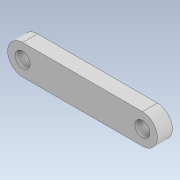
# Autodesk Inventor part: 地桿
Saved by Autodesk Inventor 2022 (Build 260153000, 153)
## iProperties
Created: 2023-05-12
Part Number: 地桿
Material: 一般
Document SubType Name: Modeling
Designer: JOU
Density: 1 g/cm^3
Appearance: 預設
Author: JOU
Autodesk Inventor part; units mm, degrees
ref_plane "YZ Plane" through (0, 0, 0) normal (1, 0, 0) x (0, 1, 0)
ref_plane "XZ Plane" through (0, 0, 0) normal (0, 1, 0) x (-1, 0, 0)
ref_plane "XY Plane" through (0, 0, 0) normal (0, 0, 1) x (1, 0, 0)
sketch "草圖1" plane through (0, 0, 0) normal (0, 0, 1) x (1, 0, 0)
  line L0 (0, 0) -> (80, 0) construction
  line L1 (0, 10) -> (80, 10)
  line L2 (80, -10) -> (0, -10)
  arc A0 (0, 10) -> (0, -10) centre (0, 0) ccw
  arc A1 (80, -10) -> (80, 10) centre (80, 0) ccw
  circle A2 centre (0, 0) radius 5
  circle A3 centre (80, 0) radius 5
  point P0 (40, 0)
  dimension "d0" = 80
  dimension "d1" = 20
  dimension "d2" = 10
  dimension "d3" = 10
  constraints: 8 end point, 4 centre point, 4 point on circle, 4 tangent, 2 coincident, 1 horizontal, 1 midpoint, 1 parallel
  measures "d0" distance of L1.start L1.end
  measures "d1" distance between parallel lines of L2 L1
  measures "d2" diameter of A2
  measures "d3" diameter of A3
extrude "擠出1" add sketch "草圖1" along normal blind 10
